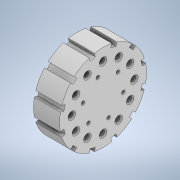
# Autodesk Inventor part: 711144 (Доделать)
Saved by Autodesk Inventor 2022 (Build 260153000, 153)
## iProperties
Created: 2021-10-22
Part Number: 711144 (Доделать)
Material: Типовые
Document SubType Name: Modeling
Designer: RaNSiD
Density: 1 g/cm^3
Appearance: По умолчанию
Author: RaNSiD
Autodesk Inventor part; units mm, degrees
ref_plane "YZ Plane" through (0, 0, 0) normal (1, 0, 0) x (0, 1, 0)
ref_plane "XZ Plane" through (0, 0, 0) normal (0, 1, 0) x (-1, 0, 0)
ref_plane "XY Plane" through (0, 0, 0) normal (0, 0, 1) x (1, 0, 0)
sketch "Эскиз1" plane through (0, 0, 0) normal (0, 0, 1) x (1, 0, 0)
  line L0 (0, 0) -> (15, 0)
  line L1 (15, 0) -> (15, 25)
  line L2 (15, 25) -> (0, 25)
  line L3 (0, 25) -> (0, 0)
  dimension "d0" = 15
  dimension "d1" = 25
  constraints: 8 end point, 2 parallel, 1 horizontal, 1 perpendicular
  measures "d0" distance of L2.end L1.end
  measures "d1" distance of L1.end L0.end
revolve "Вращение1" add sketch "Эскиз1" angle 360 about axis through (0, 0, 0) along (1, 0, 0)
sketch "Эскиз2" plane through (0, 0, 0) normal (-1, 0, 0) x (0, 0, 1)
  circle A0 centre (0, 0) radius 25 construction
  line L0 (18.7065, 16.5852) -> (17.2923, 15.1709)
  line L1 (17.2923, 15.1709) -> (15.1709, 17.2923)
  line L2 (15.1709, 17.2923) -> (16.5852, 18.7065)
  arc A1 (18.7065, 16.5852) -> (16.5852, 18.7065) centre (0, 0) ccw
  line L3 (0, 0) -> (16.2316, 16.2316) construction
  line L4 (0, 0) -> (25, 0) construction
  line L5 (0, 0) -> (21.6506, 12.5) construction
  line L6 (4.4923, 22.561) -> (5.0099, 24.4929)
  arc A2 (7.9077, 23.7164) -> (5.0099, 24.4929) centre (0, 0) ccw
  line L7 (7.9077, 23.7164) -> (7.3901, 21.7846)
  line L8 (7.3901, 21.7846) -> (4.4923, 22.561)
  line L9 (0, 0) -> (12.5, 21.6506) construction
  line L10 (-7.3901, 21.7846) -> (-7.9077, 23.7164)
  arc A3 (-5.0099, 24.4929) -> (-7.9077, 23.7164) centre (0, 0) ccw
  line L11 (-5.0099, 24.4929) -> (-4.4923, 22.561)
  line L12 (-4.4923, 22.561) -> (-7.3901, 21.7846)
  line L13 (0, 0) -> (0, 25) construction
  line L14 (-17.2923, 15.1709) -> (-18.7065, 16.5852)
  arc A4 (-16.5852, 18.7065) -> (-18.7065, 16.5852) centre (0, 0) ccw
  line L15 (-16.5852, 18.7065) -> (-15.1709, 17.2923)
  line L16 (-15.1709, 17.2923) -> (-17.2923, 15.1709)
  line L17 (0, 0) -> (-12.5, 21.6506) construction
  line L18 (-22.561, 4.4923) -> (-24.4929, 5.0099)
  arc A5 (-23.7164, 7.9077) -> (-24.4929, 5.0099) centre (0, 0) ccw
  line L19 (-23.7164, 7.9077) -> (-21.7846, 7.3901)
  line L20 (-21.7846, 7.3901) -> (-22.561, 4.4923)
  line L21 (0, 0) -> (-21.6506, 12.5) construction
  line L22 (-21.7846, -7.3901) -> (-23.7164, -7.9077)
  arc A6 (-24.4929, -5.0099) -> (-23.7164, -7.9077) centre (0, 0) ccw
  line L23 (-24.4929, -5.0099) -> (-22.561, -4.4923)
  line L24 (-22.561, -4.4923) -> (-21.7846, -7.3901)
  line L25 (0, 0) -> (-25, 0) construction
  line L26 (-15.1709, -17.2923) -> (-16.5852, -18.7065)
  arc A7 (-18.7065, -16.5852) -> (-16.5852, -18.7065) centre (0, 0) ccw
  line L27 (-18.7065, -16.5852) -> (-17.2923, -15.1709)
  line L28 (-17.2923, -15.1709) -> (-15.1709, -17.2923)
  line L29 (0, 0) -> (-21.6506, -12.5) construction
  line L30 (-4.4923, -22.561) -> (-5.0099, -24.4929)
  arc A8 (-7.9077, -23.7164) -> (-5.0099, -24.4929) centre (0, 0) ccw
  line L31 (-7.9077, -23.7164) -> (-7.3901, -21.7846)
  line L32 (-7.3901, -21.7846) -> (-4.4923, -22.561)
  line L33 (0, 0) -> (-12.5, -21.6506) construction
  line L34 (7.3901, -21.7846) -> (7.9077, -23.7164)
  arc A9 (5.0099, -24.4929) -> (7.9077, -23.7164) centre (0, 0) ccw
  line L35 (5.0099, -24.4929) -> (4.4923, -22.561)
  line L36 (4.4923, -22.561) -> (7.3901, -21.7846)
  line L37 (0, 0) -> (0, -25) construction
  line L38 (17.2923, -15.1709) -> (18.7065, -16.5852)
  arc A10 (16.5852, -18.7065) -> (18.7065, -16.5852) centre (0, 0) ccw
  line L39 (16.5852, -18.7065) -> (15.1709, -17.2923)
  line L40 (15.1709, -17.2923) -> (17.2923, -15.1709)
  line L41 (0, 0) -> (12.5, -21.6506) construction
  line L42 (22.561, -4.4923) -> (24.4929, -5.0099)
  arc A11 (23.7164, -7.9077) -> (24.4929, -5.0099) centre (0, 0) ccw
  line L43 (23.7164, -7.9077) -> (21.7846, -7.3901)
  line L44 (21.7846, -7.3901) -> (22.561, -4.4923)
  line L45 (0, 0) -> (21.6506, -12.5) construction
  line L46 (21.7846, 7.3901) -> (23.7164, 7.9077)
  arc A12 (24.4929, 5.0099) -> (23.7164, 7.9077) centre (0, 0) ccw
  line L47 (24.4929, 5.0099) -> (22.561, 4.4923)
  line L48 (22.561, 4.4923) -> (21.7846, 7.3901)
  point P0 (5.9412, 22.1728)
  point P1 (-5.9412, 22.1728)
  point P2 (-16.2316, 16.2316)
  point P3 (-22.1728, 5.9412)
  point P4 (-22.1728, -5.9412)
  point P5 (-16.2316, -16.2316)
  point P6 (-5.9412, -22.1728)
  point P7 (5.9412, -22.1728)
  point P8 (16.2316, -16.2316)
  point P9 (22.1728, -5.9412)
  point P10 (22.1728, 5.9412)
  dimension "d6" = 3
  dimension "d7" = 45
  dimension "d8" = 2
  dimension "d11" = 360
  constraints: 98 end point, 27 point on circle, 12 centre point, 2 perpendicular, 1 concentric, 1 horizontal, 1 midpoint, 1 parallel, 145 other
  measures "d6" distance between parallel lines of L2 L0
  measures "d7" angle of L4 L3
  measures "d8" distance of L0.start L0.end
extrude "Выдавливание1" cut sketch "Эскиз2" against normal through all
sketch "Эскиз3" plane through (0, 0, 0) normal (-1, 0, 0) x (0, 0, 1)
  point P0 (0, 0)
  point P1 (0, 18)
  point P2 (-9, 15.5885)
  point P3 (-15.5885, 9)
  point P4 (-18, 0)
  point P5 (-15.5885, -9)
  point P6 (-9, -15.5885)
  point P7 (0, -18)
  point P8 (9, -15.5885)
  point P9 (15.5885, -9)
  point P10 (18, 0)
  point P11 (15.5885, 9)
  point P12 (9, 15.5885)
  dimension "d15" = 18
  dimension "d18" = 360
  constraints: 1 vertical alignment, 13 other
  measures "d15" distance of point (0, 0) point (0, 18)
hole "Отверстие1" at (0, 18, 0) at (0, 15.5885, -9) at (0, 9, -15.5885) at (0, 0, -18) at (0, -9, -15.5885) at (0, -15.5885, -9) at (0, -18, 0) at (0, -15.5885, 9) at (0, -9, 15.5885) at (0, 0, 18) at (0, 9, 15.5885) at (0, 15.5885, 9) direction (1, 0, 0) diameter 3 end through all
chamfer "Фаска1" distance 0.7 angle 45 1 edges at (0, 18, -1.5)
chamfer "Фаска2" distance 0.7 angle 45 23 edges at (0, 15.5885, 7.5) (0, 9, 14.0885) (0, 15.5885, -10.5) (0, 9, -17.0885) (15, 9, -17.0885) (15, 15.5885, -10.5) (0, 0, -19.5) (15, 0, -19.5) (0, -9, -17.0885) (15, -9, -17.0885) (15, -15.5885, -10.5) (0, -15.5885, -10.5) (15, -18, -1.5) (0, -18, -1.5) (0, -15.5885, 7.5) (15, -15.5885, 7.5) (0, -9, 14.0885) (15, -9, 14.0885) (15, 0, 16.5) (0, 0, 16.5) (15, 9, 14.0885) (15, 15.5885, 7.5) (15, 18, -1.5)
sketch "Эскиз4" plane through (0, 0, 0) normal (-1, 0, 0) x (0, 0, 1)
  line L0 (7.3901, 21.7846) -> (4.4923, 22.561) construction
  line L1 (0, 0) -> (5.9412, 22.1728) construction
  line L2 (4.4923, 22.561) -> (7.3901, 21.7846) projected
  point P0 (3.1058, 11.5911)
  point P1 (-8.4853, 8.4853)
  point P2 (-11.5911, -3.1058)
  point P3 (-3.1058, -11.5911)
  point P4 (8.4853, -8.4853)
  point P5 (11.5911, 3.1058)
  dimension "d33" = 12
  dimension "d36" = 360
  constraints: 2 end point, 1 midpoint, 1 point on line, 7 other
  measures "d33" distance of L1.start point (3.106, 11.591)
hole "Отверстие2" at (0, 11.5911, 3.1058) at (0, 8.4853, -8.4853) at (0, -3.1058, -11.5911) at (0, -11.5911, -3.1058) at (0, -8.4853, 8.4853) at (0, 3.1058, 11.5911) direction (1, 0, 0) diameter 2 end through all
